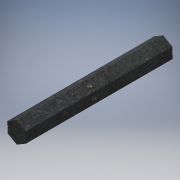
# Autodesk Inventor part: rollerwheelpoweraxel
Saved by Autodesk Inventor 2016 (Build 200138000, 138)
## iProperties
Created: 2016-01-30
Part Number: rollerwheelpoweraxel
Material: Steel
Document SubType Name: Modeling
Designer: student
Density: 7.85 g/cm^3
Appearance: Plate
Mass: 111.404 g
Surface Area: 47.4916 cm^2
Volume: 14.1916 cm^3
Author: student
Autodesk Inventor part; units mm, degrees
ref_plane "YZ Plane" through (0, 0, 0) normal (1, 0, 0) x (0, 1, 0)
ref_plane "XZ Plane" through (0, 0, 0) normal (0, 1, 0) x (-1, 0, 0)
ref_plane "XY Plane" through (0, 0, 0) normal (0, 0, 1) x (1, 0, 0)
sketch "Sketch1" plane through (0, 0, 0) normal (0, 0, 1) x (1, 0, 0)
  line L0 (6.3852, -3.6045) -> (0.071, -7.332)
  line L1 (0.071, -7.332) -> (-6.3142, -3.7275)
  line L2 (-6.3142, -3.7275) -> (-6.3852, 3.6045)
  line L3 (-6.3852, 3.6045) -> (-0.071, 7.332)
  line L4 (-0.071, 7.332) -> (6.3142, 3.7275)
  line L5 (6.3142, 3.7275) -> (6.3852, -3.6045)
  point P0 (0, 0)
  point P1 (0, 0)
  dimension "d0" = 12.7
  constraints: 12 end point, 1 coincident, 13 other
  measures "d0" distance between parallel lines of L2 L5
extrude "Extrusion1" add sketch "Sketch1" along normal blind 101.6
body "Solid1"
